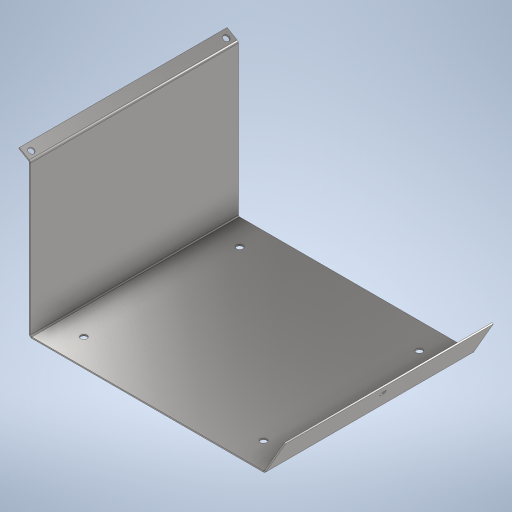
# Autodesk Inventor part: zetdeel_hoog
Saved by Autodesk Inventor 2023 (Build 270158000, 158)
## iProperties
Created: 2022-10-06
Part Number: zetdeel_hoog
Material: Steel, Galvanized
Document SubType Name: Sheet Metal
Designer: VoorL
Density: 7.85 g/cm^3
Sheet Metal Rule: Default_mm
Appearance: Galvanized
Flat Pattern Width: 33.7159 cm
Flat Pattern Length: 16 cm
Flat Pattern Area: 539.455 cm^2
Sheet Metal Width: 337,159 mm
Sheet Metal Length: 160,000 mm
Sheet Metal Area: 53945,452 mm^2
Author: VoorL
Autodesk Inventor part; units mm, degrees
ref_plane "YZ Plane" through (0, 0, 0) normal (1, 0, 0) x (0, 1, 0)
ref_plane "XZ Plane" through (0, 0, 0) normal (0, 1, 0) x (-1, 0, 0)
ref_plane "XY Plane" through (0, 0, 0) normal (0, 0, 1) x (1, 0, 0)
sketch "Sketch1" plane through (0, 0, 0) normal (0, 1, 0) x (-1, 0, 0)
  line L0 (-90.75, 80) -> (90.75, 80)
  line L1 (90.75, 80) -> (90.75, -80)
  line L2 (90.75, -80) -> (-90.75, -80)
  line L3 (-90.75, -80) -> (-90.75, 80)
  line L4 (-90.75, 80) -> (90.75, -80) construction
  line L5 (90.75, 80) -> (-90.75, -80) construction
  point P0 (0, 0)
  dimension "d0" = 181.5
  dimension "d1" = 160
  constraints: 12 end point, 2 midpoint, 2 parallel, 1 horizontal, 1 perpendicular
  measures "d0" distance of L1.end L2.end
  measures "d1" distance of L0.end L1.end
extrude "Extrusion1" add sketch "Sketch1" along normal blind 1
sketch "Sketch2" plane through (-89.75, 0, 80) normal (-1, 0, 0) x (0, -1, 0)
  line L0 (0, -160) -> (0, 0)
  line L1 (0, 0) -> (-117.5, 0)
  line L2 (-117.5, 0) -> (-117.5, -160)
  line L3 (-117.5, -160) -> (0, -160)
  constraints: 6 end point, 1 horizontal, 1 perpendicular, 1 vertical
edge flange "Flange1" height 117.5 angle 90 thickness 1 bend radius 1 thickness toward (-1, 0, 0) relief tear relief width 1 relief depth 0.5 edges at (-90.75, 1, 0) wall of the first edge with corners at (-89.75, 0, -80) (-89.75, 0, 80) (-89.75, 117.5, 80) (-89.75, 117.5, -80)
bend "Bend1"
corner "Corner1"
sketch "Sketch3" plane through (-90.25, 116.634, 80) normal (0.5, 0.8660254, 0) x (0.8660254, -0.5, 0)
  line L0 (0, -160) -> (0, 0)
  line L1 (0, 0) -> (-10, 0)
  line L2 (-10, 0) -> (-10, -160)
  line L3 (-10, -160) -> (0, -160)
  constraints: 6 end point, 1 horizontal, 1 perpendicular, 1 vertical
edge flange "Flange2" height 10 angle -60 thickness 1 bend radius 1 thickness toward (0.5, 0.8660254, 0) relief tear relief width 1 relief depth 0.5 edges at (-89.75, 117.5, 0) wall of the first edge with corners at (-90.25, 116.634, -80) (-90.25, 116.634, 80) (-98.9103, 121.634, 80) (-98.9103, 121.634, -80)
bend "Bend2"
corner "Corner2"
sketch "Sketch4" plane through (-98.4103, 122.5, 80) normal (0.5, 0.8660254, 0) x (0, 0, -1)
  line L0 (160, 0) -> (0, 0) projected
  line L1 (80, 0) -> (80, -5)
  line L2 (80, 0) -> (85, 0) construction
  line L3 (80, -5) -> (155, -5)
  line L4 (80, -5) -> (155, -5) construction
  line L5 (80, -5) -> (5, -5)
  line L6 (80, -5) -> (155, -5) construction
  point P0 (80, -146.4758)
  dimension "d25" = 5
  dimension "d26" = 90
  dimension "d27" = 75
  dimension "d28" = 0
  dimension "d29" = 75
  dimension "d30" = 180
  constraints: 12 end point, 5 horizontal, 3 equal length, 1 midpoint, 1 vertical
  measures "d25" distance of L1.start L1.end
  measures "d26" angle of L1 L2
  measures "d27" distance of L1.end L3.end
  measures "d28" distance between parallel lines of L3 L4
  measures "d29" distance of L1.end L5.end
  measures "d30" angle of L5 L6
hole "Hole1" at (-94.0801, 120, 75) at (-94.0801, 120, -75) direction (-0.5, -0.8660254, 0) diameter 4.5 depth 1 tip angle 118
sketch "Sketch5" plane through (89.884, 0.5, -80) normal (0.8660254, -0.5, 0) x (0.5, 0.8660254, 0)
  line L0 (0, 160) -> (0, 0)
  line L1 (0, 0) -> (31.5, 0)
  line L2 (31.5, 0) -> (31.5, 160)
  line L3 (31.5, 160) -> (0, 160)
  constraints: 6 end point, 1 horizontal, 1 perpendicular, 1 vertical
edge flange "Flange3" height 31.5 angle 60 thickness 1 bend radius 1 thickness toward (0.8660254, -0.5, 0) relief tear relief width 1 relief depth 0.5 edges at (90.75, 1, 0) wall of the first edge with corners at (89.884, 0.5, 80) (89.884, 0.5, -80) (105.634, 27.7798, -80) (105.634, 27.7798, 80)
bend "Bend3"
corner "Corner3"
sketch "Sketch6" plane through (106.5, 27.2798, 80) normal (0.8660254, -0.5, 0) x (0, 0, -1)
  line L0 (0, 0) -> (160, 0) projected
  line L1 (80, 0) -> (80, -10)
  line L2 (80, 0) -> (90, 0) construction
  point P0 (80, -76.875)
  dimension "d48" = 10
  dimension "d49" = 90
  constraints: 4 end point, 1 horizontal, 1 midpoint, 1 perpendicular, 1 vertical
  measures "d48" distance of L1.start L1.end
  measures "d49" angle of L1 L2
hole "Hole3" at (101.5, 18.6195, 0) direction (-0.8660254, 0.5, 0) diameter 4.5 depth 1 tip angle 118
sketch "Sketch7" plane through (0, 0, 0) normal (0, -1, 0) x (1, 0, 0)
  line L0 (89.5953, -80) -> (89.5953, 80) projected
  line L1 (-88.75, 80) -> (89.5953, 80) projected
  line L2 (-88.75, 80) -> (-88.75, -80) projected
  line L3 (89.5953, -80) -> (-88.75, -80) projected
  line L4 (-88.75, 80) -> (-68.75, 80)
  line L5 (-88.75, 80) -> (89.5953, 80) projected
  line L6 (-68.75, 80) -> (-68.75, 60)
  line L7 (-88.75, 0) -> (89.5953, 0)
  line L8 (0.4226, 80) -> (0.4226, -80)
  point P0 (0, 0)
  point P1 (-68.75, -60)
  point P2 (69.5953, 60)
  point P3 (69.5953, -60)
  dimension "d67" = 20
  dimension "d68" = 20
  constraints: 8 end point, 4 midpoint, 3 symmetric about line, 1 perpendicular, 1 point on line
  measures "d67" distance of L1.start L4.end
  measures "d68" distance of L4.end L6.end
hole "Hole4" at (69.5953, 0, -60) at (-68.75, 0, -60) at (-68.75, 0, 60) at (69.5953, 0, 60) direction (0, 1, 0) diameter 5 depth 1 tip angle 118
equation "\"d36\" = Thickness"
equation "\"d65\" = Thickness"
equation "\"d74\" = Thickness"
equation "\"d4\" = Thickness"
equation "\"d5\" = BendReliefWidth"
equation "\"d6\" = BendReliefDepth"
equation "\"d7\" = MinimumRemnant"
equation "\"d8\" = TransitionRadius"
equation "\"d11\" = BendRadius"
equation "\"d12\" = CornerReliefSize"
equation "\"d13\" = GapSize"
equation "\"d14\" = JacobiRadiusSize"
equation "\"d15\" = BendReliefWidth"
equation "\"d16\" = BendReliefDepth"
equation "\"d17\" = MinimumRemnant"
equation "\"d18\" = TransitionRadius"
equation "\"d21\" = BendRadius"
equation "\"d22\" = CornerReliefSize"
equation "\"d23\" = GapSize"
equation "\"d24\" = JacobiRadiusSize"
equation "\"d38\" = BendReliefWidth"
equation "\"d39\" = BendReliefDepth"
equation "\"d40\" = MinimumRemnant"
equation "\"d41\" = TransitionRadius"
equation "\"d44\" = BendRadius"
equation "\"d45\" = CornerReliefSize"
equation "\"d46\" = GapSize"
equation "\"d47\" = JacobiRadiusSize"
equation "\"BendRadius\" = Thickness"
equation "\"BendReliefWidth\" = Thickness"
equation "\"BendReliefDepth\" = 0.5 * Thickness"
equation "\"CornerReliefSize\" = 4 * Thickness"
equation "\"MinimumRemnant\" = 2 * Thickness"
equation "\"TransitionRadius\" = BendRadius"
equation "\"JacobiRadiusSize\" = BendRadius"
equation "\"GapSize\" = Thickness"
equation "\"Thickness\" = 1"
body "Solid1"
